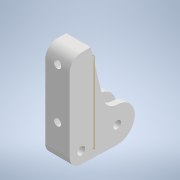
# Autodesk Inventor part: Motor Pressure Lever
Saved by Autodesk Inventor 2022.2 (Build 262287000, 287)
## iProperties
Created: 2022-08-15
Part Number: Motor Pressure Lever
Material: Generic
Document SubType Name: Modeling
Designer: Ilewicz
Density: 1 g/cm^3
Appearance: Default
Author: Ilewicz
Autodesk Inventor part; units mm, degrees
ref_plane "YZ Plane" through (0, 0, 0) normal (1, 0, 0) x (0, 1, 0)
ref_plane "XZ Plane" through (0, 0, 0) normal (0, 1, 0) x (-1, 0, 0)
ref_plane "XY Plane" through (0, 0, 0) normal (0, 0, 1) x (1, 0, 0)
derived "Motor.ipt"
sketch "Sketch1" plane through (0, 0, 0) normal (1, 0, 0) x (0, 1, 0)
  circle A0 centre (0, 0) radius 8 construction
  circle A1 centre (-2, 15.5) radius 1.65
  arc A2 (-2, 20.5) -> (-6.9974, 15.6616) centre (-2, 15.5) ccw
  arc A3 (-7.4961, 0.2424) -> (7.4966, -0.2254) centre (0, 0) ccw
  line L0 (12.6265, 6.1122) -> (34.65, 11.5)
  line L1 (-7.4961, 0.2424) -> (-6.9974, 15.6616)
  circle A4 centre (0, 0) radius 1.65
  arc A5 (12.6265, 6.1122) -> (7.4966, -0.2254) centre (14.2264, -0.4278) ccw
  line L2 (7.5, 0) -> (23.5407, 0)
  line L3 (-2, 20.5) -> (29.65, 20.5)
  arc A6 (34.65, 15.5) -> (29.65, 20.5) centre (29.65, 15.5) ccw
  line L4 (34.65, 15.5) -> (34.65, 11.5)
  line L5 (34.65, 11.5) -> (34.65, 11.5)
  line L6 (34.65, -2.5) -> (34.65, 3.5) projected
  point P0 (-7.4013, 1.2126)
  point P1 (-1.9895, -7.2313)
  dimension "d0" = 16
  dimension "d1" = 3.3
  dimension "d3" = 15.5
  dimension "d4" = 2
  dimension "d6" = 5
  dimension "d7" = 15
  dimension "d8" = 3.3
  dimension "d35" = 4
  constraints: 14 point on circle, 12 end point, 7 centre point, 7 tangent, 4 coincident, 2 horizontal, 2 point on line, 1 collinear, 1 equal radius, 1 perpendicular, 1 vertical
  measures "d0" diameter of A0
  measures "d1" diameter of A1
  measures "d3" vertical distance of A1.centre point (0, 0)
  measures "d4" horizontal distance of point (0, 0) A1.centre
  measures "d6" radius of A2
  measures "d7" diameter of A3
  measures "d8" diameter of A4
  measures "d35" distance from line of L5 A1.centre
extrude "Extrusion1" add sketch "Sketch1" along normal blind 2.5
sketch "Sketch2" plane through (2.5, 0, 0) normal (1, 0, 0) x (0, 0, -1)
  circle A0 centre (0, 0) radius 8.2
  line L0 (-6.1122, 12.6265) -> (-11.5, 34.65) projected
  arc A1 (-20.5, -2) -> (-15.6616, -6.9974) centre (-15.5, -2) ccw projected
  line L1 (-15.6616, -6.9974) -> (-0.2424, -7.4961) projected
  arc A2 (-0.2424, -7.4961) -> (0.2254, 7.4966) centre (0, 0) ccw projected
  circle A3 centre (-15.5, -2) radius 1.65 projected
  circle A4 centre (0, 0) radius 1.65 projected
  arc A5 (-6.1122, 12.6265) -> (0.2254, 7.4966) centre (0.4278, 14.2264) ccw projected
  line L2 (-20.5, 29.65) -> (-20.5, -2) projected
  line L3 (-11.5, 34.65) -> (-15.5, 34.65) projected
  arc A6 (-15.5, 34.65) -> (-20.5, 29.65) centre (-15.5, 29.65) ccw projected
  point P0 (-4.8811, 6.589)
  point P1 (-2.0091, 7.9501)
  point P2 (8.2, 0)
  point P3 (-3.2278, 7.538)
  point P4 (-3.5558, -7.3889)
  point P5 (-0.638, -8.1751)
  constraints: 1 centre point, 1 coincident
extrude "Extrusion2" add sketch "Sketch2" along normal blind 5.5 contours A0 L1 A1 L2 A6 L3 L0 A5
sketch "Sketch3" plane through (8, 0, 0) normal (1, 0, 0) x (0, 0, -1)
  arc A0 (-2.0091, 7.9501) -> (-3.5558, -7.3889) centre (0, 0) ccw projected
  arc A1 (-6.1122, 12.6265) -> (-2.0091, 7.9501) centre (0.4278, 14.2264) ccw projected
  line L0 (-6.1122, 12.6265) -> (-11.5, 34.65) projected
  arc A2 (-20.5, -2) -> (-15.6616, -6.9974) centre (-15.5, -2) ccw projected
  line L1 (-15.6616, -6.9974) -> (-3.5558, -7.3889) projected
  circle A3 centre (-15.5, -2) radius 1.65 projected
  circle A4 centre (0, 0) radius 1.65 projected
  arc A5 (-2.0091, 7.9501) -> (-3.5558, -7.3889) centre (0, 0) ccw projected
  arc A6 (-0.2424, -7.4961) -> (0.2254, 7.4966) centre (0, 0) ccw projected
  line L2 (-11.5, 34.65) -> (-15.5, 34.65) projected
  arc A7 (-15.5, 34.65) -> (-20.5, 29.65) centre (-15.5, 29.65) ccw projected
  line L3 (-20.5, 29.65) -> (-20.5, -2) projected
  line L4 (-3.5558, -7.3889) -> (-0.2424, -7.4961) projected
  arc A8 (-2.0091, 7.9501) -> (0.2254, 7.4966) centre (0.4278, 14.2264) ccw projected
  point P0 (-3.2278, 7.538)
  point P1 (-0.638, -8.1751)
  point P2 (-3.2278, 7.538)
  point P3 (-3.5558, -7.3889)
  point P4 (-2.0091, 7.9501)
extrude "Extrusion3" add sketch "Sketch3" along normal blind 2.5
ref_plane "Work Plane1" through (5.25, 0, 0) normal (1, 0, 0) x (0, 0, -1)
sketch "Sketch5" plane through (5.25, 0, 0) normal (1, 0, 0) x (0, 0, -1)
  line L0 (-24.9072, 8.5441) -> (34.3598, 8.5441)
  point P0 (0, 0)
  constraints: 2 end point, 1 horizontal
sketch "Sketch6" plane through (0, 5.1162, 0) normal (0, 0, -1) x (-1, 0, 0)
  point P0 (0, -5.1162)
  point P1 (-5.25, 3.4279)
  point P2 (-5.25, 3.4279)
  point P3 (-5.25, 3.4279)
  point P4 (-5.25, 3.4279)
  constraints: 1 coincident
hole "Hole1" at (5.25, 8.5441, 0) direction (0, 0, 1) diameter 3 end through all countersink diameter 4 countersink angle 90
fillet "Fillet1" radius 2 3 edges at (6.6544, 9.0712, 3.9028) (3.8456, 9.071, 3.9027) (5.2495, 7.0441, 4.1977)
sketch "Sketch7" plane through (0, -2, 20.5) normal (0, 0, 1) x (1, 0, 0)
  line L0 (10.5, 1.65) -> (10.5, -1.65) projected
  circle A0 centre (5.25, 32) radius 1.5
  line L1 (5.25, 45.08) -> (5.25, -13.93) projected
  point P0 (0, 2)
  point P1 (10.5, 0)
  dimension "d37" = 3
  dimension "d39" = 32
  constraints: 1 centre point, 1 midpoint, 1 point on line
  measures "d37" diameter of A0
  measures "d39" vertical distance of A0.centre point (10.5, 0)
extrude "Extrusion5" cut sketch "Sketch7" against normal through all
ref_plane "Work Plane2" through (0, -2, 10.5) normal (0, 0, 1) x (1, 0, 0)
sketch "Sketch9" plane through (0, -2, 10.5) normal (0, 0, 1) x (1, 0, 0)
  circle A0 centre (5.25, 32) radius 1.5 projected
  line L0 (5.25, 36.1569) -> (8.85, 34.0785)
  line L1 (8.85, 34.0785) -> (8.85, 29.9215)
  line L2 (8.85, 29.9215) -> (5.25, 27.8431)
  line L3 (5.25, 27.8431) -> (1.65, 29.9215)
  line L4 (1.65, 29.9215) -> (1.65, 34.0785)
  line L5 (1.65, 34.0785) -> (5.25, 36.1569)
  point P0 (0, 2)
  dimension "d43" = 7.2
  constraints: 12 end point, 1 coincident, 13 other
  measures "d43" distance between parallel lines of L1 L4
extrude "Extrusion6" cut sketch "Sketch9" along normal mid plane 4
equation "\"d3\" = 0.5 * x_hole"
equation "\"x_hole\" = 31.000011"
body "Solid1"
